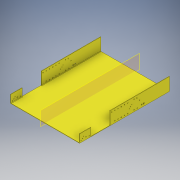
# Autodesk Inventor part: SheetBottomFloor
Saved by Autodesk Inventor 2019 (Build 230136000, 136)
## iProperties
Created: 2016-02-09
Part Number: SheetBottomFloor
Material: Aluminum 6061
Document SubType Name: Sheet Metal
Designer: steele
Density: 2.7 g/cm^3
Appearance: Canary
Mass: 4353.07 g
Surface Area: 10287.7 cm^2
Volume: 1612.25 cm^3
Flat Pattern Width: 54.61 cm
Flat Pattern Length: 71.12 cm
Flat Pattern Area: 3883.86 cm^2
Sheet Metal Rule: Default_mm
Sheet Metal Width: 21.500 in
Sheet Metal Length: 28.000 in
Sheet Metal Area: 602.000 in^2
Author: steele
Autodesk Inventor part; units mm, degrees
ref_plane "XZ Plane" through (0, 0, 0) normal (0, 1, 0) x (-1, 0, 0)
ref_plane "XY Plane" through (0, 0, 0) normal (0, 0, 1) x (1, 0, 0)
sketch "Sketch1" plane through (0, 0, 0) normal (0, 0, 1) x (1, 0, 0)
  line L0 (0, 0) -> (-273.05, 0)
  line L1 (-273.05, 0) -> (-273.05, 101.6)
  line L2 (-273.05, 101.6) -> (-269.875, 101.6)
  line L3 (-269.875, 101.6) -> (-269.875, 3.175)
  line L4 (0, 0) -> (0, 3.175) construction
  line L5 (0, 3.175) -> (-269.875, 3.175)
  line L6 (0, 0) -> (273.05, 0)
  line L7 (273.05, 0) -> (273.05, 101.6)
  line L8 (273.05, 101.6) -> (269.875, 101.6)
  line L9 (269.875, 101.6) -> (269.875, 3.175)
  line L10 (0, 3.175) -> (269.875, 3.175)
  dimension "d0" = 101.6
  dimension "d1" = 273.05
  dimension "d2" = 3.175
  dimension "d4" = 3.175
  constraints: 22 end point, 4 symmetric about line, 2 horizontal, 2 perpendicular, 1 parallel, 1 vertical
  measures "d0" distance of L0.end L1.end
  measures "d1" distance of L0.start L0.end
  measures "d2" distance between parallel lines of L1 L3
  measures "d4" distance of L0.start L4.end
extrude "Extrusion1" add sketch "Sketch1" along normal mid plane 711.2
fillet "Fillet1" radius 3.175 2 edges at (-269.875, 3.175, 0) (269.875, 3.175, 0)
sketch "Sketch5" plane through (-269.875, 101.6, 355.6) normal (1, 0, 0) x (0, 0, -1)
  circle A0 centre (12.7, -34.925) radius 2.5527 projected
  circle A1 centre (22.225, -25.4) radius 2.5527 projected
  circle A2 centre (31.75, -15.875) radius 2.5527 projected
  circle A3 centre (50.8, -15.875) radius 3.3782 projected
  circle A4 centre (76.2, -15.875) radius 3.7287 projected
  circle A5 centre (12.7, -88.9) radius 2.667 projected
  circle A6 centre (22.225, -79.375) radius 2.667 projected
  circle A7 centre (31.75, -69.85) radius 2.5527 projected
  circle A8 centre (50.8, -82.55) radius 3.8164 projected
  circle A9 centre (76.2, -88.9) radius 3.3782 projected
  circle A10 centre (101.4806, -93.6752) radius 3.3782 projected
  circle A11 centre (212.631, -93.6752) radius 3.3782 projected
  circle A12 centre (228.6, -88.9) radius 3.7287 projected
  circle A13 centre (279.4, -86.36) radius 3.8164 projected
  circle A14 centre (228.6, -15.875) radius 3.3782 projected
  circle A15 centre (254, -15.875) radius 3.7287 projected
  circle A16 centre (279.4, -15.875) radius 3.3782 projected
  circle A17 centre (304.8, -15.875) radius 3.3782 projected
  circle A18 centre (330.2, -15.875) radius 3.7287 projected
  circle A19 centre (355.6, -15.875) radius 3.3782 projected
  circle A20 centre (381, -15.875) radius 3.3782 projected
  circle A21 centre (431.8, -15.875) radius 3.7287 projected
  circle A22 centre (454.025, -19.05) radius 3.8164 projected
  circle A23 centre (508, -82.55) radius 3.8164 projected
  circle A24 centre (457.2, -88.9) radius 3.3782 projected
  circle A25 centre (431.8, -88.9) radius 3.7287 projected
  circle A26 centre (475.0995, -43.8435) radius 3.3782 projected
  circle A27 centre (412.75, -42.8625) radius 2.5527 projected
  circle A28 centre (403.225, -52.3875) radius 2.667 projected
  circle A29 centre (393.7, -61.9125) radius 2.5527 projected
  circle A30 centre (381, -88.9) radius 3.3782 projected
  circle A31 centre (355.6, -88.9) radius 3.3782 projected
  circle A32 centre (330.2, -88.9) radius 3.7287 projected
  circle A33 centre (304.8, -88.9) radius 3.3782 projected
  circle A34 centre (492.125, -82.55) radius 4.826 projected
  circle A35 centre (508, -82.55) radius 5.2255 projected
  point P0 (355.6, -101.6)
extrude "Extrusion5" cut sketch "Sketch5" along normal through all both and the other way through all
sketch "Sketch12" plane through (-269.875, 19.05, -152.4) normal (1, 0, 0) x (0, 0, -1)
  circle A0 centre (0, 0) radius 4.2111
  point P0 (-152.4, -19.05)
  constraints: 1 centre point
extrude "Extrusion10" cut sketch "Sketch12" along normal through all both and the other way through all
sketch "Sketch25" plane through (-273.05, 0, 355.6) normal (-1, 0, 0) x (0, 0, 1)
  line L0 (-711.2, 3.175) -> (0, 3.175) projected
  line L1 (0, 101.6) -> (-711.2, 101.6) projected
  line L2 (-241.3, 3.175) -> (-88.9, 3.175)
  line L3 (-88.9, 3.175) -> (-88.9, 63.5)
  line L4 (-88.9, 101.6) -> (-241.3, 101.6)
  line L5 (-241.3, 101.6) -> (-241.3, 3.175)
  line L6 (0, 101.6) -> (0, 0) projected
  line L7 (0, 101.6) -> (-88.9, 101.6)
  line L8 (-88.9, 63.5) -> (0, 63.5)
  line L9 (0, 63.5) -> (0, 101.6)
  point P0 (-355.6, 0)
  dimension "d81" = 88.9
  dimension "d82" = 241.3
  dimension "d83" = 38.1
  constraints: 14 end point, 3 parallel, 2 horizontal, 2 point on line, 1 perpendicular
  measures "d81" distance between parallel lines of L3 L6
  measures "d82" distance between parallel lines of L5 L6
  measures "d83" distance between parallel lines of L8 L1
extrude "Extrusion22" cut sketch "Sketch25" against normal through all contours L5 L1 L6 L8 L3 L0
equation "\"BendRadius\" = Thickness"
equation "\"BendReliefWidth\" = Thickness"
equation "\"BendReliefDepth\" = 0.5 * Thickness"
equation "\"CornerReliefSize\" = 4 * Thickness"
equation "\"MinimumRemnant\" = 2 * Thickness"
equation "\"TransitionRadius\" = BendRadius"
equation "\"JacobiRadiusSize\" = BendRadius"
equation "\"GapSize\" = Thickness"
equation "\"Thickness\" = 3.175"
body "Solid1"
